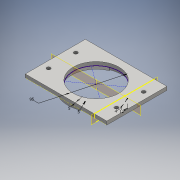
# Autodesk Inventor part: AZ100 ASI LX-4000 stage adapter
Saved by Autodesk Inventor 2016 (Build 200138000, 138)
## iProperties
Created: 2015-08-14
Part Number: AZ100 ASI LX-4000 stage adapter
Material: Generic
Document SubType Name: Modeling
Designer: kthorn
Density: 1 g/cm^3
Appearance: Default
Author: kthorn
Autodesk Inventor part; units mm, degrees
ref_plane "YZ Plane" through (0, 0, 0) normal (1, 0, 0) x (0, 1, 0)
ref_plane "XZ Plane" through (0, 0, 0) normal (0, 1, 0) x (-1, 0, 0)
ref_plane "XY Plane" through (0, 0, 0) normal (0, 0, 1) x (1, 0, 0)
sketch "Sketch1" plane through (0, 0, 0) normal (0, 0, 1) x (1, 0, 0)
  line L0 (14.4686, 36.4073) -> (141.0686, 36.4073) construction
  line L1 (141.0686, 36.4073) -> (141.0686, -14.2927) construction
  line L2 (141.0686, -14.2927) -> (14.4686, -14.2927) construction
  line L3 (14.4686, -14.2927) -> (14.4686, 36.4073) construction
  circle A0 centre (14.4686, 36.4073) radius 3.375
  circle A1 centre (14.4686, -14.2927) radius 3.375
  circle A2 centre (141.0686, -14.2927) radius 3.375
  circle A3 centre (141.0686, 36.4073) radius 3.375
  line L4 (1.7686, 67.0573) -> (153.7686, 67.0573)
  line L5 (153.7686, 67.0573) -> (153.7686, -44.9427)
  line L6 (153.7686, -44.9427) -> (1.7686, -44.9427)
  line L7 (1.7686, -44.9427) -> (1.7686, 67.0573)
  line L8 (14.4686, 36.4073) -> (1.7686, 67.0573) construction
  line L9 (14.4686, -14.2927) -> (1.7686, -44.9427) construction
  line L10 (141.0686, -14.2927) -> (153.7686, -44.9427) construction
  line L11 (141.0686, 36.4073) -> (153.7686, 67.0573) construction
  line L12 (153.7686, 11.0573) -> (1.7686, 11.0573) construction
  point P0 (0, 0)
  dimension "d1" = 126.6
  dimension "d2" = 50.7
  dimension "d3" = 6.75
  dimension "d4" = 152
  dimension "d5" = 112
  constraints: 26 end point, 4 centre point, 4 coincident, 4 parallel, 3 equal radius, 2 equal length, 2 horizontal, 2 midpoint, 2 perpendicular
  measures "d1" distance of L0.start L0.end
  measures "d2" distance of L2.end L0.start
  measures "d3" diameter of A3
  measures "d4" distance of L4.start L4.end
  measures "d5" distance of L6.end L4.start
extrude "Extrusion1" add sketch "Sketch1" along normal blind 6.5
sketch "Sketch4" plane through (0, 0, 0) normal (0, 0, -1) x (-1, 0, 0)
  circle A0 centre (-77.7686, 11.0573) radius 47.5
  line L0 (-153.7686, 67.0573) -> (-1.7686, 67.0573) construction
  line L1 (-1.7686, -44.9427) -> (-153.7686, -44.9427) construction
  line L2 (-1.7686, 67.0573) -> (-153.7686, -44.9427) construction
  line L3 (-1.7686, -44.9427) -> (-153.7686, 67.0573) construction
  circle A1 centre (-77.7686, 11.0573) radius 52.5
  circle A2 centre (-77.7686, 11.0573) radius 42.5
  point P0 (0, 0)
  dimension "d12" = 95
  dimension "d13" = 5
  dimension "d34" = 5
  constraints: 4 end point, 3 centre point, 3 coincident, 1 midpoint
  measures "d12" diameter of A0
  measures "d13" radial gap between concentric circles of A1 A0
  measures "d34" radial gap between concentric circles of A0 A2
extrude "Extrusion2" add sketch "Sketch4" along normal blind 8 contours A1
ref_plane "Work Plane3" through (1.7686, 11.0573, 0) normal (0, -1, 0) x (1, 0, 0)
sketch "Sketch6" plane through (1.7686, 11.0573, 0) normal (0, -1, 0) x (1, 0, 0)
  line L0 (28.5, 0) -> (28.5, -8) projected
  line L1 (123.5, -8) -> (28.5, -8) projected
  line L2 (28.5, -8) -> (30.5, -8)
  line L3 (30.5, -8) -> (28.5, -1)
  line L4 (28.5, -8) -> (28.5, -1)
  line L5 (76, -10.9) -> (76, 9.4) projected
  dimension "d16" = 2
  dimension "d17" = 7
  constraints: 6 end point, 2 point on line, 1 collinear
  measures "d16" distance of L1.end L2.end
  measures "d17" distance of L1.end L3.end
revolve "Revolution1" add sketch "Sketch6" angle 135 mid plane about axis through (77.7686, 11.0573, -8) along (0, 0, 1)
ref_plane "Work Plane4" through (130.2686, 11.0573, 0) normal (1, 0, 0) x (0, 1, 0)
sketch "Sketch7" plane through (130.2686, 11.0573, 0) normal (1, 0, 0) x (0, 1, 0)
  line L0 (-52.5, -8) -> (52.5, -8) projected
  line L1 (56, 0) -> (-56, 0) projected
  line L2 (56, 0) -> (56, 6.5) projected
  line L3 (-56, 6.5) -> (56, 6.5) projected
  line L4 (-56, 0) -> (-56, 6.5) projected
  line L5 (47.5, -8) -> (-47.5, -8) projected
  line L6 (-47.5, 0) -> (47.5, 0) projected
  line L7 (6, -8) -> (-6, -8)
  line L8 (-6, -8) -> (-6, 0)
  line L9 (-6, 0) -> (6, 0)
  line L10 (6, 0) -> (6, -8)
  line L11 (0, -10.9) -> (0, 9.4) projected
  circle A0 centre (0, -4) radius 2
  point P0 (-11.0573, 0)
  point P1 (-43.8843, -8)
  point P2 (43.8843, -8)
  point P3 (0, -8)
  dimension "d23" = 12
  dimension "d24" = 4
  constraints: 8 end point, 4 point on line, 2 parallel, 1 centre point, 1 horizontal, 1 midpoint, 1 perpendicular
  measures "d23" distance between parallel lines of L8 L10
  measures "d24" diameter of A0
extrude "Extrusion3" add sketch "Sketch7" against normal up to next contours L8 L1 L11 A0 L0 | L11 A0 L1 L10 L0
extrude "Extrusion4" add sketch "Sketch7" along normal blind 0.5 contours L8 L1 L11 A0 L0 | L11 A0 L1 L10 L0
extrude "Extrusion5" cut sketch "Sketch7" against normal up to next contours A0 L11 | L11 A0
chamfer "Chamfer1" distance 2 angle 45 4 edges at (11.0936, -14.2927, 0) (11.0936, 36.4073, 0) (137.6936, 36.4073, 0) (137.6936, -14.2927, 0)
extrude "Extrusion6" cut sketch "Sketch4" against normal through all contours A2
body "Solid1"
